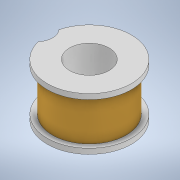
# Autodesk Inventor part: Катушка
Saved by Autodesk Inventor 2022 (Build 260153000, 153)
## iProperties
Created: 2024-04-28
Part Number: Катушка
Material: Типовые
Document SubType Name: Modeling
Designer: Pavel
Density: 1 g/cm^3
Appearance: По умолчанию
Author: Pavel
Autodesk Inventor part; units mm, degrees
ref_plane "YZ Plane" through (0, 0, 0) normal (1, 0, 0) x (0, 1, 0)
ref_plane "XZ Plane" through (0, 0, 0) normal (0, 1, 0) x (-1, 0, 0)
ref_plane "XY Plane" through (0, 0, 0) normal (0, 0, 1) x (1, 0, 0)
sketch "Эскиз1" plane through (0, 0, 0) normal (1, 0, 0) x (0, 1, 0)
  line L0 (0, 0) -> (0, 3.75) construction
  line L1 (0, 3.75) -> (0, 8)
  line L2 (0, 8) -> (1, 8)
  line L3 (1, 8) -> (1, 4.75)
  line L4 (1, 4.75) -> (9, 4.75)
  line L5 (9, 4.75) -> (9, 8)
  line L6 (9, 8) -> (10, 8)
  line L7 (10, 8) -> (10, 3.75)
  line L8 (10, 3.75) -> (0, 3.75)
  line L9 (13.294, 0) -> (-4.7382, 0) construction
  dimension "d0" = 3.75
  dimension "d1" = 4.25
  dimension "d2" = 1
  dimension "d3" = 3.25
  dimension "d4" = 8
  dimension "d5" = 1
  dimension "d6" = 4.25
  constraints: 20 end point, 6 perpendicular, 2 horizontal, 2 vertical
  measures "d0" distance of L0.start L0.end
  measures "d1" distance of L0.end L1.end
  measures "d2" distance of L1.end L2.end
  measures "d3" distance of L2.end L3.end
  measures "d4" distance of L3.end L4.end
  measures "d5" distance of L5.end L6.end
  measures "d6" distance of L6.end L7.end
revolve "Вращение1" add sketch "Эскиз1" angle 360 about axis through (0, 13.294, 0) along (0, -1, 0)
sketch "Эскиз2" plane through (0, 10, 0) normal (0, 1, 0) x (1, 0, 0)
  line L0 (0, 0) -> (-10, 0) construction
  circle A0 centre (-10, 0) radius 3
  dimension "d8" = 10
  dimension "d9" = 6
  constraints: 2 end point, 1 centre point, 1 coincident, 1 horizontal
  measures "d8" distance of L0.start L0.end
  measures "d9" diameter of A0
extrude "Выдавливание1" cut sketch "Эскиз2" against normal blind 10
sketch "Эскиз3" plane through (0, 1, 0) normal (0, 1, 0) x (1, 0, 0)
  circle A0 centre (0, 0) radius 7
  circle A1 centre (0, 0) radius 4.75
  dimension "d12" = 14
  constraints: 2 centre point, 2 coincident
  measures "d12" diameter of A0
extrude "Выдавливание2" add sketch "Эскиз3" along normal blind 8 separate body
